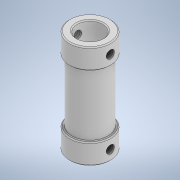
# Autodesk Inventor part: Khop_Noi_Truc_5_5
Saved by Autodesk Inventor 2022 (Build 260153000, 153)
## iProperties
Created: 2022-11-18
Part Number: Khop_Noi_Truc_5_5
Material: Generic
Document SubType Name: Modeling
Designer: nguye
Density: 1 g/cm^3
Appearance: Default
Author: nguye
Autodesk Inventor part; units mm, degrees
ref_plane "XZ Plane" through (0, 0, 0) normal (0, 1, 0) x (-1, 0, 0)
sketch "Sketch1" plane through (0, 0, 0) normal (0, 1, 0) x (-1, 0, 0)
  circle A0 centre (0, 0) radius 2.5
  circle A1 centre (0, 0) radius 4
  dimension "d0" = 5
  dimension "d1" = 8
  constraints: 2 centre point, 2 coincident
  measures "d0" diameter of A0
  measures "d1" diameter of A1
extrude "Extrusion1" add sketch "Sketch1" along normal blind 20
ref_plane "Work Plane1" through (0, 10, 0) normal (0, 1, 0) x (1, 0, 0)
sketch "Sketch2" plane through (0, 10, 0) normal (0, 1, 0) x (1, 0, 0)
  circle A0 centre (0, 0) radius 2.5
  circle A1 centre (0, 0) radius 4 projected
  circle A2 centre (0, 0) radius 3.5
  dimension "d5" = 5
  dimension "d6" = 7
  constraints: 2 centre point, 2 coincident
  measures "d5" diameter of A0
  measures "d6" diameter of A2
extrude "Extrusion2" cut sketch "Sketch2" along normal mid plane 12 contours A1
chamfer "Chamfer1" distance 0.2 angle 45 4 edges at (4, 0, 0) (4, 4, 0) (4, 16, 0) (4, 20, 0)
chamfer "Chamfer2" distance 0.2 angle 45 2 edges at (2.5, 20, 0) (2.5, 0, 0)
ref_plane "Work Plane2" through (4, 0, 0) normal (1, 0, 0) x (0, 1, 0)
sketch "Sketch3" plane through (4, 0, 0) normal (1, 0, 0) x (0, 1, 0)
  point P0 (0, 0)
  point P1 (2, 0)
  point P2 (18, 0)
  dimension "d15" = 16
  dimension "d16" = 2
  constraints: 2 horizontal alignment
  measures "d15" distance of point (18, 0) point (2, 0)
  measures "d16" distance of point (0, 0) point (2, 0)
hole "Hole1" at (4, 2, 0) at (4, 18, 0) direction (-1, 0, 0) diameter 1.567 end through all thread size "M2x0.4" class "6H" standard "ISO Metric profile"
body "Solid1"
